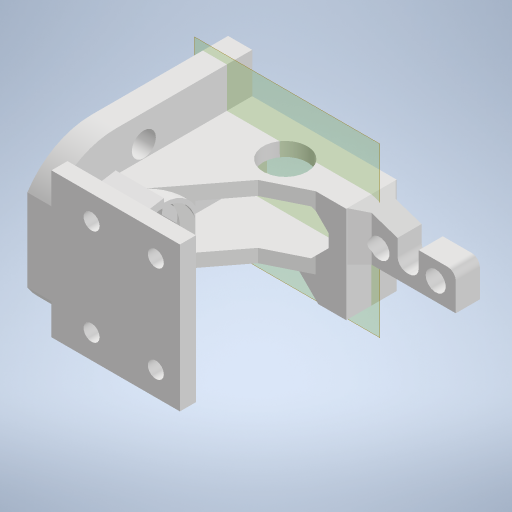
# Autodesk Inventor part: крепежная основа
Saved by Autodesk Inventor 2024.2 (Build 282272000, 272)
## iProperties
Created: 2026-02-10
Part Number: крепежная основа
Material: Типовые
Document SubType Name: Modeling
Designer: Service
Density: 1 g/cm^3
Appearance: По умолчанию
Author: Service
Autodesk Inventor part; units mm, degrees
ref_plane "YZ Plane" through (0, 0, 0) normal (1, 0, 0) x (0, 1, 0)
ref_plane "XZ Plane" through (0, 0, 0) normal (0, 1, 0) x (-1, 0, 0)
ref_plane "XY Plane" through (0, 0, 0) normal (0, 0, 1) x (1, 0, 0)
sketch "Эскиз1" plane through (0, 0, 0) normal (1, 0, 0) x (0, 1, 0)
  line L0 (-7.4467, -2.3641) -> (2.5533, -2.3641)
  circle A0 centre (-2.4467, 2.6685) radius 4
  line L1 (2.5533, 8.6685) -> (6.5533, 8.6685)
  line L2 (6.5533, 8.6685) -> (6.5533, 10.6685)
  line L3 (6.5533, 10.6685) -> (-11.4467, 10.6685)
  line L4 (-11.4467, 10.6685) -> (-11.4467, 8.6685)
  line L5 (-11.4467, 8.6685) -> (-7.4467, 8.6685)
  line L6 (-7.4467, -2.3641) -> (-7.4467, 2.6685)
  line L7 (2.5533, -2.3641) -> (2.5533, 2.6685)
  line L8 (2.5533, 8.6685) -> (1.5533, 8.6685)
  line L9 (-7.4467, 8.6685) -> (-6.4467, 8.6685)
  line L10 (-6.4467, 8.6685) -> (-7.4467, 2.6685)
  line L11 (1.5533, 8.6685) -> (2.5533, 2.6685)
  line L12 (2.5533, 2.6685) -> (2.0533, -2.3641)
  line L13 (-7.4467, 2.6685) -> (-6.4467, -2.3641)
  circle A1 centre (-2.4467, 2.6685) radius 4.5
  line L14 (2.5533, 2.6685) -> (2.0533, 2.6685)
  line L15 (-7.4467, 2.6685) -> (-6.9467, 2.6685)
  point P0 (0, 0)
  dimension "d0" = 8
  dimension "d4" = 4
  dimension "d5" = 4
  dimension "d7" = 10
  dimension "d8" = 2
  dimension "d9" = 8
  dimension "d14" = 1
  dimension "d15" = 1
  dimension "d39" = 9
  constraints: 32 end point, 5 point on line, 3 horizontal, 3 perpendicular, 2 centre point, 2 point on circle, 2 vertical, 1 coincident
  measures "d0" diameter of A0
  measures "d4" distance of L1.start L1.end
  measures "d5" distance of L4.end L5.end
  measures "d7" distance of L0.start L0.end
  measures "d8" distance of L3.end L4.end
  measures "d9" distance from line of A0.centre L3
  measures "d14" distance of L1.start L8.end
  measures "d15" distance of L5.end L9.end
  measures "d39" diameter of A1
extrude "Выдавливание1" add sketch "Эскиз1" along normal blind 6 contours L10 L9 L5 L4 L3 L2 L1 L8 L11 L14 A1 L15 | A1
sketch "Эскиз2" plane through (0, -11.4467, 10.6685) normal (0, 0, 1) x (1, 0, 0)
  circle A0 centre (13, 15) radius 1
  circle A1 centre (13, 3) radius 1
  line L0 (6, 13) -> (6, 5) projected
  circle A2 centre (5, 15) radius 1
  circle A3 centre (5, 3) radius 1
  line L1 (6, 18) -> (6, 0) projected
  line L2 (0, 0) -> (6, 0) projected
  point P0 (0, 11.4467)
  dimension "d10" = 12
  dimension "d11" = 2
  dimension "d12" = 2
  dimension "d22" = 2
  dimension "d25" = 12
  dimension "d26" = 2
  dimension "d27" = 2
  dimension "d28" = 8
  dimension "d31" = 8
  dimension "d32" = 3
  dimension "d42" = 1
  dimension "d43" = 1
  constraints: 4 centre point
  measures "d10" distance of A1.centre A0.centre
  measures "d11" diameter of A1
  measures "d12" diameter of A0
  measures "d22" vertical distance of L0.start A0.centre
  measures "d25" distance of A3.centre A2.centre
  measures "d26" diameter of A3
  measures "d27" diameter of A2
  measures "d28" distance of A3.centre A1.centre
  measures "d31" distance of A0.centre A2.centre
  measures "d32" distance from line of L2 A3.centre
  measures "d42" horizontal distance of L0.end A3.centre
  measures "d43" distance from line of L1 A2.centre
sketch "Эскиз3" plane through (0, 0, 0) normal (-1, 0, 0) x (0, 0, 1)
  line L0 (8.6685, 6.5533) -> (10.6685, 6.5533) projected
  line L1 (8.6685, 1.5533) -> (8.6685, 6.5533) projected
  line L2 (2.6685, 2.5533) -> (8.6685, 1.5533) projected
  line L3 (8.6685, -6.4467) -> (2.6685, -7.4467) projected
  line L4 (8.6685, -11.4467) -> (8.6685, -6.4467) projected
  line L5 (10.6685, -11.4467) -> (8.6685, -11.4467) projected
  line L6 (10.6685, 6.5533) -> (10.6685, -11.4467) projected
  circle A0 centre (2.6685, -2.4467) radius 4 projected
  circle A1 centre (2.6685, -2.4467) radius 9.5
  line L7 (2.6685, -2.4467) -> (-2.0922, -10.6677)
  line L8 (2.6685, -2.4467) -> (-2.0922, 5.7744)
  line L9 (2.6685, -2.4467) -> (12.1685, -2.4467)
  circle A2 centre (-0.8394, -8.5043) radius 1.5
  circle A3 centre (-0.8394, 3.611) radius 1.5
  line L10 (2.6685, -7.4467) -> (2.6685, -6.9467) projected
  line L11 (2.6685, 2.0533) -> (2.6685, 2.5533) projected
  arc A4 (2.6685, 2.0533) -> (2.6685, -6.9467) centre (2.6685, -2.4467) ccw projected
  point P0 (0, 0)
  point P1 (10.6685, -7.5701)
  point P2 (10.6685, 2.6768)
  dimension "d33" = 19
  dimension "d34" = 3
  dimension "d35" = 2.5
  dimension "d36" = 2.5
  constraints: 6 end point, 3 centre point, 3 point on circle, 2 point on line, 1 coincident, 1 equal radius
  measures "d33" diameter of A1
  measures "d34" diameter of A3
  measures "d35" distance of L7.end A2.centre
  measures "d36" distance of L8.end A3.centre
extrude "Выдавливание3" add sketch "Эскиз3" along normal blind 3 contours A1 L6 L9 A0 L8 A4 L11 L2 L1 | L1 L2 L11 A4 L8 A3 A1 | L8 A3 A4 L7 A2 A1 | L6 A1 L4 L3 L10 A4 L7 A0 L9 | L7 A2 A4 L10 L3 L4 A1 | A0 L7 A4 L8
sketch "Эскиз4" plane through (6, 0, 0) normal (1, 0, 0) x (0, 0, -1)
  line L0 (-8.6685, 1.5533) -> (-8.6685, 6.5533) projected
  line L1 (-10.6685, 6.5533) -> (-10.6685, -11.4467) projected
  line L2 (-8.6685, -11.4467) -> (-8.6685, -6.4467) projected
  line L3 (-10.6685, 6.5533) -> (-8.6685, 6.5533)
  line L4 (-8.6685, 6.5533) -> (-8.6685, -11.4467)
  line L5 (-8.6685, -11.4467) -> (-10.6685, -11.4467)
  line L6 (-10.6685, -11.4467) -> (-10.6685, 6.5533)
  point P0 (0, 0)
  constraints: 8 end point, 2 parallel, 1 horizontal, 1 perpendicular
extrude "Выдавливание4" add sketch "Эскиз4" along normal blind 10
extrude "Выдавливание2" cut sketch "Эскиз2" against normal through all
ref_plane "РабПлоскость2" through (0, -2.4467, -14.3315) normal (0, 0, -1) x (-1, 0, 0)
ref_plane "РабПлоскость1" through (0, -2.4467, -1.3315) normal (0, 0, -1) x (-1, 0, 0)
sketch "Эскиз5" plane through (0, -2.4467, -14.3315) normal (0, 0, -1) x (-1, 0, 0)
  line L0 (0, 9.5) -> (3, 9.5) projected
  line L1 (3, 9.5) -> (0, 9.5)
  line L2 (0, 9.5) -> (3, 9.5) projected
  line L3 (0, 5) -> (0, 4) projected
  line L4 (0, 4.5) -> (0, 9.5)
  line L5 (0, 4.5) -> (-12, 4.5)
  line L6 (3, 9.5) -> (3, -9.4711)
  line L7 (3, -9.4711) -> (0, -9.4711)
  line L8 (0, -9.4711) -> (0, -4.4835)
  line L9 (0, -4.4835) -> (-12, -4.4835)
  line L10 (-12, -4.4835) -> (-12, 4.5)
  line L11 (-3, 4.5) -> (-3, -4.4835)
  point P0 (-16, -9)
  point P1 (-6, 4.5)
  dimension "d107" = 12
  dimension "d108" = 3
  constraints: 18 end point, 4 perpendicular, 4 point on line, 1 collinear, 1 horizontal, 1 midpoint, 1 parallel, 1 vertical
  measures "d107" distance of L8.end L9.end
  measures "d108" distance of L6.end L7.end
extrude "Выдавливание5" add sketch "Эскиз5" against normal up to next contours L0 L6 L7 L8 L9 L11 L5 L3 L4
ref_plane "РабПлоскость4" through (16, -6.9301, -14.3315) normal (1, 0, 0) x (0, 0, -1)
ref_plane "РабПлоскость5" through (16, -6.9467, -14.2858) normal (0.7935674, 0, 0.6084824) x (0, 1, 0)
sketch "Эскиз16" plane through (16, -6.9467, -14.2858) normal (0.7935674, 0, 0.6084824) x (0, 1, 0)
  ellipse E0 centre (4.5, 21.3646) end of major axis (9, 21.3646) minor radius 3.5711 (0.0165, 21.0587) -> (9, 21.3646) ccw projected
  line L0 (9, 21.3646) -> (9, 7.874)
  line L1 (0.0165, 21.0587) -> (0.0165, 7.874)
  line L2 (0.0165, 7.874) -> (9, 7.874)
  line L3 (9, 7.874) -> (0.0165, 7.874) projected
  point P0 (6.9467, 21.0725)
  constraints: 6 end point, 3 vertical, 1 collinear, 1 perpendicular, 1 other
extrude "Выдавливание14" add sketch "Эскиз16" against normal up to next
ref_plane "РабПлоскость6" through (18, 0, 0) normal (1, 0, 0) x (0, 0, -1)
sketch "Эскиз17" plane through (18, 0, 0) normal (1, 0, 0) x (0, 0, -1)
  line L0 (8.0373, 2.0533) -> (14.3315, 2.0533) projected
  line L1 (8.0373, 2.0533) -> (14.3315, 2.0533)
  line L2 (14.3315, 2.0533) -> (14.3315, -6.9301)
  line L3 (8.0373, -6.9301) -> (8.0373, 2.0533)
  line L4 (8.0373, -6.9301) -> (14.3315, -6.9301) projected
  line L5 (8.0373, -6.9301) -> (8.0373, -9.9597)
  line L6 (8.0373, -9.9597) -> (14.3315, -9.9597)
  line L7 (14.3315, -9.9597) -> (14.3315, -6.9301)
  point P0 (0, 0)
  dimension "d138" = 3.0296
  constraints: 12 end point, 3 perpendicular, 1 horizontal, 1 vertical
  measures "d138" distance between parallel lines of L4 L6
extrude "Выдавливание15" add sketch "Эскиз17" against normal up to next contours L0 L2 L4 L3
chamfer "Фаска6" distance 3 angle 45 1 edges at (11.2088, -2.4384, -8.0373)
sketch "Эскиз18" plane through (0, -2.4467, -14.3315) normal (0, 0, -1) x (-1, 0, 0)
  line L0 (-15.8286, 2.7687) -> (-1.8286, 2.7687)
  line L1 (-1.8286, 2.7687) -> (-1.8286, -2.8313)
  line L2 (-1.8286, -2.8313) -> (-15.8286, -2.8313)
  line L3 (-15.8286, -2.8313) -> (-15.8286, 2.7687)
  point P0 (0, 2.4467)
  dimension "d120" = 14
  dimension "d121" = 5.6
  constraints: 8 end point, 2 parallel, 1 horizontal, 1 perpendicular
  measures "d120" distance of L1.end L2.end
  measures "d121" distance of L0.end L1.end
extrude "Выдавливание16" cut sketch "Эскиз18" against normal up to surface (13.0875 mm away)
chamfer "Фаска7" distance 2 angle 45 2 edges at (15.8286, 0.322, -11.1844) (15.8286, -5.278, -11.1844)
sketch "Эскиз19" plane through (0, 2.0533, 2.6685) normal (0, 1, 0) x (1, 0, 0)
  circle A0 centre (8.8286, 12.2909) radius 2.75
  point P0 (0, 2.6685)
  point P1 (1.8286, 17)
  dimension "d127" = 5.5
  dimension "d128" = 7
  constraints: 1 centre point
  measures "d127" diameter of A0
  measures "d128" horizontal distance of point (1.829, 17) A0.centre
extrude "Выдавливание17" cut sketch "Эскиз19" against normal up to surface (1.7313 mm away)
extrude "Выдавливание18" add sketch "Эскиз17" against normal blind 5 contours L4 L7 L6 L5
chamfer "Фаска8" distance 1.514 angle 45 2 edges at (13, -9.9597, -11.1844) (13, -6.9301, -11.1844)
sketch "Эскиз23" plane through (0, -2.4467, -14.3315) normal (0, 0, -1) x (-1, 0, 0)
  point P0 (0, 2.4467)
ref_plane "РабПлоскость7" through (0, -2.4467, -11.1844) normal (0, 0, -1) x (-1, 0, 0)
sketch "Эскиз24" plane through (0, -2.4467, -11.1844) normal (0, 0, -1) x (-1, 0, 0)
  line L0 (-30, -1.5911) -> (-18, -1.5911) projected
  line L1 (-18, -1.5911) -> (-18, 1.9089) projected
  arc A0 (-18, 1.9089) -> (-19, 2.9089) centre (-19, 1.9089) ccw projected
  line L2 (-19, 2.9089) -> (-22.75, 2.9089) projected
  line L3 (-22.75, 2.9089) -> (-22.75, 0.9089) projected
  arc A1 (-24.0186, -0.2892) -> (-22.75, 0.9089) centre (-23.95, 0.9089) ccw projected
  line L4 (-24.0186, -0.2892) -> (-24.1186, -0.2892) projected
  arc A2 (-25.3872, 0.9089) -> (-24.1186, -0.2892) centre (-24.1872, 0.9089) ccw projected
  line L5 (-25.3872, 0.9089) -> (-25.3872, 2.9089) projected
  line L6 (-25.3872, 2.9089) -> (-29, 2.9089) projected
  arc A3 (-29, 2.9089) -> (-30, 1.9089) centre (-29, 1.9089) ccw projected
  line L7 (-30, 1.9089) -> (-30, -1.5911) projected
  circle A4 centre (-27.5, 0.6589) radius 1.25 projected
  circle A5 centre (-20.5, 0.6589) radius 1.25 projected
  line L8 (0, 4.5) -> (-18, 4.5) projected
  line L9 (-22.75, 2.9089) -> (-18, 4.5)
  line L10 (-18, 4.5) -> (-18, 1.9089)
  point P0 (0, 2.4467)
  constraints: 4 end point, 1 vertical
extrude "Выдавливание20" add sketch "Эскиз24" along normal mid plane 3
chamfer "Фаска9" distance 1.515 angle 45 2 edges at (18, -0.9922, -9.6844) (18, -0.9922, -12.6844)
sketch "Эскиз11" plane through (12.4836, -6.9467, -1.3315) normal (1, 0, 0) x (0, 0, -1)
  line L0 (-10, 13.5) -> (-12, 13.5) projected
  line L1 (-12, -4.5) -> (-10, -4.5) projected
  line L2 (-12, 13.5) -> (-10, 13.5)
  line L3 (-10, 13.5) -> (-10, -4.5)
  line L4 (-10, -4.5) -> (-12, -4.5)
  line L5 (-12, -4.5) -> (-12, 13.5)
  point P0 (-1.3315, 6.9467)
  point P1 (-12, -4.5)
  constraints: 8 end point, 2 parallel, 1 horizontal, 1 perpendicular
sketch "Эскиз8" plane through (0, -2.4467, -14.3315) normal (0, 0, -1) x (-1, 0, 0)
  line L0 (-12.4836, 3) -> (-4.4836, 3)
  line L1 (-4.4836, 3) -> (-4.4836, -3)
  line L2 (-4.4836, -3) -> (-12.4836, -3)
  line L3 (-12.4836, -3) -> (-12.4836, 3)
  line L4 (-12.4836, 4.5) -> (-12.4836, -4.5) projected
  line L5 (0, 4.5) -> (-12.4836, 4.5) projected
  point P0 (0, 2.4467)
  point P1 (-8.4836, 3)
  dimension "d76" = 8
  dimension "d77" = 6
  dimension "d78" = 1.5
  constraints: 8 end point, 2 parallel, 1 collinear, 1 horizontal, 1 midpoint, 1 perpendicular
  measures "d76" distance of L1.end L2.end
  measures "d77" distance of L0.end L1.end
  measures "d78" distance from line of L5 point (-8.484, 3)
sketch "Эскиз12" plane through (0, 2.0533, -14.3315) normal (0, 1, 0) x (1, 0, 0)
  line L0 (0, 0) -> (0, -17) projected
  line L1 (0, -25) -> (23.4836, -25) projected
  circle A0 centre (5, -7) radius 2.5
  line L2 (-3, 0) -> (-3, -17) projected
  point P0 (0, -14.3315)
  dimension "d94" = 5
  dimension "d95" = 8
  dimension "d96" = 18
  constraints: 1 centre point
  measures "d94" diameter of A0
  measures "d95" distance from line of L2 A0.centre
  measures "d96" distance from line of L1 A0.centre
sketch "Эскиз13" plane through (0, 2.6768, 10.6685) normal (0, 0, 1) x (1, 0, 0)
  line L0 (0, 3.8765) -> (16, 3.8765) projected
  line L1 (0, 3.8765) -> (0, 0) projected
  line L2 (0, 0) -> (-3, 0) projected
  line L3 (-3, -10.247) -> (-3, 0) projected
  line L4 (0, -10.247) -> (-3, -10.247) projected
  line L5 (0, -10.247) -> (0, -14.1235) projected
  line L6 (0, -14.1235) -> (16, -14.1235) projected
  circle A0 centre (5, -11.1235) radius 1 projected
  circle A1 centre (5, 0.8765) radius 1 projected
  circle A2 centre (13, 0.8765) radius 1
  circle A3 centre (13, -11.1235) radius 1
  line L7 (16, 3.8765) -> (16, -14.1235) projected
  point P0 (0, -2.6768)
  dimension "d99" = 2
  dimension "d100" = 2
  dimension "d101" = 8
  dimension "d102" = 8
  dimension "d103" = 12
  dimension "d104" = 3
  constraints: 2 centre point
  measures "d99" diameter of A2
  measures "d100" diameter of A3
  measures "d101" distance of A0.centre A3.centre
  measures "d102" distance of A1.centre A2.centre
  measures "d103" distance of A3.centre A2.centre
  measures "d104" distance from line of L0 A2.centre
